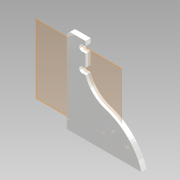
# Autodesk Inventor part: CFHoneycomb
Saved by Autodesk Inventor 2021 (Build 250183000, 183)
## iProperties
Created: 2020-11-23
Part Number: CFHoneycomb
Material: ABS Plastic
Document SubType Name: Modeling
Designer: Kanenas
Mass: 5.05227 g
Surface Area: 36.7766 cm^2
Volume: 4.76629 cm^3
Density: 1.06 g/cm^3
Appearance: Smooth - White
Author: Kanenas
Autodesk Inventor part; units mm, degrees
ref_plane "YZ Plane" through (0, 0, 0) normal (1, 0, 0) x (0, 1, 0)
ref_plane "XZ Plane" through (0, 0, 0) normal (0, 1, 0) x (-1, 0, 0)
sketch "Sketch1" plane through (0, 0, 0) normal (0, 0, 1) x (1, 0, 0)
  line L0 (-6, 27.5) -> (6, 27.5)
  line L1 (6, 27.5) -> (6, -27.5)
  line L2 (6, -27.5) -> (-6, -27.5)
  line L3 (-6, -27.5) -> (-6, 27.5)
  line L4 (-6, 27.5) -> (6, -27.5) construction
  line L5 (6, 27.5) -> (-6, -27.5) construction
  line L6 (6, -27.5) -> (46, -27.5)
  line L7 (46, -27.5) -> (46, -6.5)
  line L8 (46, -6.5) -> (6, -6.5)
  line L9 (6, -6.5) -> (6, -27.5)
  point P0 (0, 0)
  point P1 (6, -6.5)
  dimension "d0" = 12
  dimension "d1" = 55
  dimension "d18" = 40
  dimension "d19" = 21
  constraints: 20 end point, 4 parallel, 2 horizontal, 2 midpoint, 2 perpendicular
  measures "d0" distance of L0.start L0.end
  measures "d1" distance of L0.end L1.end
  measures "d18" distance of L1.end L6.end
  measures "d19" distance of L6.end L7.end
extrude "Extrusion1" add sketch "Sketch1" along normal mid plane 3.3
sketch "Sketch2" plane through (0, 0, 1.65) normal (0, 0, 1) x (1, 0, 0)
  circle A0 centre (6, 22.5) radius 2.05
  circle A1 centre (6, 10.5) radius 2.05
  line L0 (6, 22.5) -> (6, 10.5) construction
  line L1 (6, 10.5) -> (6, 22.5)
  line L2 (-6, 27.5) -> (-6, -27.5) projected
  line L3 (7.5, -30) -> (-6, -30) projected
  line L4 (6, -6.5) -> (6, 27.5) projected
  line L5 (-6, -27.5) -> (46, -27.5) projected
  line L6 (3.95, 24.55) -> (6, 24.55)
  line L7 (6, 24.55) -> (6, 20.45)
  line L8 (6, 20.45) -> (3.95, 20.45)
  line L9 (6, 12.55) -> (3.95, 12.55)
  line L10 (3.95, 8.45) -> (6, 8.45)
  line L11 (6, 8.45) -> (6, 12.55)
  circle A2 centre (3.95, 22.5) radius 2.05
  circle A3 centre (3.95, 10.5) radius 2.05
  point P0 (0, 0)
  point P1 (4.975, 8.7246)
  point P2 (4.975, 12.2754)
  point P3 (4.975, 20.7246)
  point P4 (4.975, 24.2754)
  dimension "d4" = 4.1
  dimension "d7" = 4.1
  dimension "d20" = 0
  dimension "d22" = 38
  dimension "d25" = 12
  constraints: 16 end point, 10 tangent, 4 centre point, 4 point on circle, 3 equal length, 2 collinear, 2 horizontal, 1 perpendicular, 1 vertical
  measures "d4" diameter of A0
  measures "d7" diameter of A1
  measures "d20" distance from line of L0.start L4
  measures "d22" distance from line of L5 L0.end
  measures "d25" distance of L0.start L0.end
extrude "Extrusion2" cut sketch "Sketch2" against normal blind 3.3 contours A0 L1 L4 | L4 A2 A0 | A0 A2 L1 | A2 A0 | A0 A2 | A1 L4 L1 | L1 A3 A1 | A1 A3 L4 | A3 A1 | A1 A3
fillet "Fillet2" radius 3 1 edges at (-6, 27.5, 0)
fillet "Fillet3" radius 10 1 edges at (46, -6.5, 0)
fillet "Fillet4" radius 45 1 edges at (6, -6.5, 0)
fillet "Fillet5" radius 1 21 edges at (-5.1213, 26.6213, 1.65) (1.5, 27.5, 1.65) (-6, -1.5, 1.65) (-6, -1.5, -1.65) (1.5, 27.5, -1.65) (-5.1213, 26.6213, -1.65) (43.2989, -9.6644, 1.65) (46, -22, 1.65) (19.8537, -2.0533, 1.65) (43.2989, -9.6644, -1.65) (46, -22, -1.65) (19.8537, -2.0533, -1.65) (6, 16.5, 1.65) (6, 16.5, -1.65) (6, 26.025, -1.65) (6, 26.025, 1.65) (6, 27.5, 0) (6, 24.55, 0) (6, 20.45, 0) (6, 8.45, 0) (6, 12.55, 0)
sketch "Sketch7" plane through (0, 0, 1.65) normal (0, 0, 1) x (1, 0, 0)
  circle A0 centre (7.0062, -4.2944) radius 3.5
  circle A1 centre (20.0062, -10.2944) radius 3.5
  circle A2 centre (34.0062, -13.2944) radius 3.5
  point P0 (0, 0)
  dimension "d29" = 7
  dimension "d30" = 7
  dimension "d31" = 7
  dimension "d32" = 6
  dimension "d33" = 3
  dimension "d34" = 13
  dimension "d35" = 14
  constraints: 3 centre point
  measures "d29" diameter of A0
  measures "d30" diameter of A1
  measures "d31" diameter of A2
  measures "d32" vertical distance of A1.centre A0.centre
  measures "d33" vertical distance of A1.centre A2.centre
  measures "d34" horizontal distance of A1.centre A0.centre
  measures "d35" horizontal distance of A2.centre A1.centre
extrude "Extrusion3" cut sketch "Sketch7" against normal blind 10
fillet "Fillet6" radius 1.5 6 edges at (3.5062, -4.2944, 1.65) (16.5062, -10.2944, 1.65) (30.5062, -13.2944, 1.65) (30.5062, -13.2944, -1.65) (16.5062, -10.2944, -1.65) (3.5062, -4.2944, -1.65)
body "Solid1"
